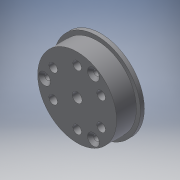
# Autodesk Inventor part: carrier_cover_13.792
Saved by Autodesk Inventor 2019.4 (Build 234330000, 330)
## iProperties
Created: 2019-06-21
Part Number: carrier_cover_13.792
Material: Generic
Document SubType Name: Modeling
Designer: cdi
Density: 1 g/cm^3
Appearance: Default
Author: cdi
Autodesk Inventor part; units mm, degrees
ref_plane "YZ Plane" through (0, 0, 0) normal (1, 0, 0) x (0, 1, 0)
ref_plane "XZ Plane" through (0, 0, 0) normal (0, 1, 0) x (-1, 0, 0)
ref_plane "XY Plane" through (0, 0, 0) normal (0, 0, 1) x (1, 0, 0)
sketch "Sketch1" plane through (0, 0, 0) normal (0, 0, 1) x (1, 0, 0)
  circle A0 centre (0, 0) radius 22
  circle A1 centre (0, 0) radius 2.5
  dimension "d0" = 44
  dimension "d1" = 5
  constraints: 2 centre point, 2 coincident
  measures "d0" diameter of A0
  measures "d1" diameter of A1
extrude "Extrusion1" add sketch "Sketch1" along normal blind 12
sketch "Sketch2" plane through (0, 0, 0) normal (0, 0, -1) x (-1, 0, 0)
  circle A0 centre (0, 0) radius 14.344
  circle A1 centre (-14.344, 0) radius 3
  dimension "d4" = 28.688
  dimension "d5" = 6
  constraints: 1 centre point, 1 coincident, 1 horizontal alignment, 2 other
  measures "d5" diameter of A1
extrude "Extrusion2" add sketch "Sketch2" along normal blind 1 contours A1 A0 | A0 A1 picked at (-13.3207, 0) picked at (-15.3207, 0)
sketch "Sketch3" plane through (14.344, 0, -1) normal (0, 0, -1) x (-1, 0, 0)
  circle A0 centre (0, 0) radius 1.55
  point P0 (14.344, 0)
  dimension "d8" = 3.1
  constraints: 1 centre point
  measures "d8" diameter of A0
extrude "Extrusion3" cut sketch "Sketch3" against normal blind 8.5
fillet "Fillet1" radius 1 1 edges at (17.344, 0, 0)
pattern_circular "Circular Pattern1" count 3 over 360 about axis through (0, 0, 0) along (0, 0, 1) of "Extrusion2", "Extrusion3", "Fillet1"
sketch "Sketch4" plane through (0, 0, 12) normal (0, 0, 1) x (1, 0, 0)
  circle A0 centre (0, 0) radius 16.5
  circle A1 centre (-16.5, 0) radius 1.5
  line L0 (0, 0) -> (-23.5834, 0)
  dimension "d15" = 33
  dimension "d16" = 3
  dimension "d27" = 23.5834
  dimension "d28" = 0
  constraints: 2 end point, 1 centre point, 1 coincident, 1 horizontal, 1 horizontal alignment, 2 other
  measures "d16" diameter of A1
  measures "d27" distance of L0.start L0.end
  measures "d28" distance from line of A1.centre L0
hole "Hole1" at (-16.5, 0, 12) direction (0, 0, -1) diameter 3 end through all countersink diameter 6 countersink angle 90
pattern_circular "Circular Pattern2" count 3 over 360 about axis through (0, 0, 0) along (0, 0, 1) of "Hole1"
sketch "Sketch5" plane through (0, 0, 12) normal (0, 0, 1) x (1, 0, 0)
  circle A0 centre (0, 0) radius 14
  circle A1 centre (0, 14) radius 2
  circle A2 centre (-12.1244, 7) radius 2
  circle A3 centre (-12.1244, -7) radius 2
  circle A4 centre (0, -14) radius 2
  circle A5 centre (12.1244, -7) radius 2
  circle A6 centre (12.1244, 7) radius 2
  dimension "d29" = 28
  dimension "d30" = 4
  dimension "d33" = 360
  constraints: 6 centre point, 1 coincident, 1 vertical alignment, 15 other
  measures "d30" diameter of A1
hole "Hole2" at (-12.1244, 7, 12) at (-12.1244, -7, 12) at (0, -14, 12) at (12.1244, -7, 12) at (0, 14, 12) at (12.1244, 7, 12) direction (0, 0, -1) diameter 3.88 end through all countersink diameter 4.34 countersink angle 7
sketch "Sketch6" plane through (0, 0, 12) normal (0, 0, 1) x (1, 0, 0)
  circle A0 centre (0, 0) radius 19.96
  circle A1 centre (0, 0) radius 27.6965
  dimension "d42" = 39.92
  constraints: 2 centre point, 2 coincident
  measures "d42" diameter of A0
extrude "Extrusion4" cut sketch "Sketch6" against normal blind 10
sketch "Sketch7" plane through (0, 0, 0) normal (0, 0, -1) x (-1, 0, 0)
  circle A0 centre (0, 0) radius 9
  dimension "d45" = 18
  constraints: 1 centre point, 1 coincident
  measures "d45" diameter of A0
extrude "Extrusion5" cut sketch "Sketch7" against normal blind 4
body "Solid1"
